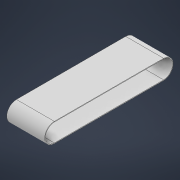
# Autodesk Inventor part: Лента конвейера
Saved by Autodesk Inventor 2022 (Build 260153000, 153)
## iProperties
Created: 2023-02-18
Part Number: Лента конвейера
Material: Типовые
Document SubType Name: Modeling
Designer: Глеб
Density: 1 g/cm^3
Appearance: По умолчанию
Author: Глеб
Autodesk Inventor part; units mm, degrees
ref_plane "YZ Plane" through (0, 0, 0) normal (1, 0, 0) x (0, 1, 0)
ref_plane "XZ Plane" through (0, 0, 0) normal (0, 1, 0) x (-1, 0, 0)
ref_plane "XY Plane" through (0, 0, 0) normal (0, 0, 1) x (1, 0, 0)
sketch "Эскиз1" plane through (0, 0, 0) normal (1, 0, 0) x (0, 1, 0)
  line L0 (-15, 100) -> (15, 100)
  line L1 (15, 100) -> (15, -100)
  line L2 (15, -100) -> (-15, -100)
  line L3 (-15, -100) -> (-15, 100)
  line L4 (-21, 0) -> (21, 0) construction
  line L5 (0, -140) -> (0, 140) construction
  point P0 (0, 0)
  dimension "d0" = 200
  dimension "d1" = 30
  constraints: 8 end point, 2 parallel, 1 horizontal, 1 perpendicular, 2 other
  measures "d0" distance of L0.end L1.end
  measures "d1" distance between parallel lines of L3 L1
extrude "Выдавливание2" add sketch "Эскиз1" along normal mid plane 59
fillet "Сопряжение1" radius 15 4 edges at (0, 15, 100) (0, -15, 100) (0, 15, -100) (0, -15, -100)
sketch "Эскиз2" plane through (29.5, 0, 0) normal (1, 0, 0) x (0, 0, -1)
  arc A0 (85, -15) -> (85, 15) centre (85, 0) ccw construction
  line L0 (85, 15) -> (-85, 15) construction
  arc A1 (-85, 15) -> (-85, -15) centre (-85, 0) ccw construction
  line L1 (-85, -15) -> (85, -15) construction
  line L2 (-99, -14) -> (99, -14)
  line L3 (99, -14) -> (99, 14)
  line L4 (99, 14) -> (-99, 14)
  line L5 (-99, 14) -> (-99, -14)
  arc A2 (-85, 14) -> (-99, 0) centre (-85, 0) ccw
  arc A3 (-85, 15) -> (-85, -15) centre (-85, 0) ccw projected
  arc A4 (-99, 0) -> (-85, -14) centre (-85, 0) ccw
  arc A5 (99, 0) -> (85, 14) centre (85, 0) ccw
  arc A6 (85, -15) -> (85, 15) centre (85, 0) ccw projected
  arc A7 (85, -14) -> (99, 0) centre (85, 0) ccw
  point P0 (0, 0)
  dimension "d11" = 198
  dimension "d12" = 28
  dimension "d13" = 1
  dimension "d14" = 1
  constraints: 8 end point, 8 point on circle, 4 centre point, 4 concentric, 4 point on line, 2 midpoint, 2 parallel, 1 horizontal, 1 perpendicular
  measures "d11" distance of L3.end L4.end
  measures "d12" distance of L4.end L2.start
  measures "d13" distance between parallel lines of L1 L2
  measures "d14" distance edge to line of A1 L5
extrude "Выдавливание3" cut sketch "Эскиз2" against normal blind 59 contours A4 A2 L4 A5 A7 L2
